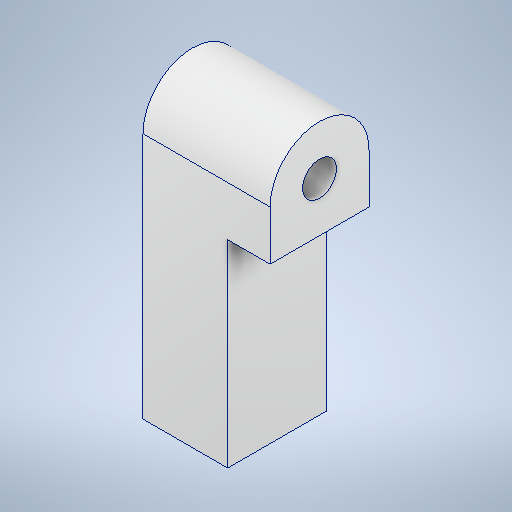
# Autodesk Inventor part: Molde
Saved by Autodesk Inventor 2025.1 (Build 291241000, 241)
## iProperties
Created: 2025-01-29
Part Number: Molde
Material: Aluminum 6061
Document SubType Name: Modeling
Designer: yovan
Mass: 51855.9 g
Surface Area: 6273.43 cm^2
Volume: 19205.9 cm^3
Density: 2.7 g/cm^3
Appearance: Aluminum - Flat
Author: yovan
Autodesk Inventor part; units mm, degrees
ref_plane "YZ Plane" through (0, 0, 0) normal (1, 0, 0) x (0, 1, 0)
ref_plane "XZ Plane" through (0, 0, 0) normal (0, 1, 0) x (-1, 0, 0)
ref_plane "XY Plane" through (0, 0, 0) normal (0, 0, 1) x (1, 0, 0)
sketch "Sketch10" plane through (0, 0, 0) normal (1, 0, 0) x (0, 1, 0)
  line L0 (0, 0) -> (175, 0)
  line L1 (350, -175) -> (350, -175)
  line L2 (175, -350) -> (0, -350)
  line L3 (0, -350) -> (0, 0)
  arc A0 (350, -175) -> (175, 0) centre (175, -175) ccw
  arc A1 (175, -350) -> (350, -175) centre (175, -175) ccw
  point P0 (350, -350)
  point P1 (350, 0)
  dimension "d73" = 350
  dimension "d74" = 350
  dimension "d76" = 175
  constraints: 8 end point, 4 point on circle, 4 point on line, 4 tangent, 2 centre point, 2 parallel, 1 concentric, 1 horizontal, 1 perpendicular
  measures "d73" distance of point (350, -350) L2.end
  measures "d74" distance of point (350, 0) point (350, -350)
  measures "d76" radius of A0
extrude "Extrusion19" add sketch "Sketch10" along normal blind 300
sketch "Sketch11" plane through (300, 0, 0) normal (1, 0, 0) x (0, 0, -1)
  arc A0 (350, 175) -> (0, 175) centre (175, 175) ccw projected
  circle A1 centre (175, 175) radius 60
  point P0 (0, 0)
  dimension "d79" = 120
  constraints: 1 centre point, 1 coincident
  measures "d79" diameter of A1
extrude "Extrusion20" cut sketch "Sketch11" against normal blind 300
sketch "Sketch12" plane through (0, 0, -350) normal (0, -1, 0) x (1, 0, 0)
  line L0 (300, 0) -> (300, 350) projected
  line L1 (0, 350) -> (300, 350)
  line L2 (300, 350) -> (300, 0)
  line L3 (300, 0) -> (0, 0)
  line L4 (0, 0) -> (0, 350)
  constraints: 8 end point, 2 parallel, 1 horizontal, 1 perpendicular
extrude "Extrusion21" add sketch "Sketch12" along normal blind 700
sketch "Sketch13" plane through (300, 0, 0) normal (1, 0, 0) x (0, 0, -1)
  circle A0 centre (175, 175) radius 60 projected
  arc A1 (350, 175) -> (0, 175) centre (175, 175) ccw projected
  arc A2 (350, 175) -> (0, 175) centre (175, 175) ccw
  line L0 (350, 175) -> (350, 0)
  line L1 (350, 0) -> (0, 0)
  line L2 (0, 0) -> (0, 175)
  circle A3 centre (175, 175) radius 60
  constraints: 6 end point, 3 point on circle, 2 centre point, 2 coincident, 1 concentric, 1 parallel
extrude "Extrusion22" add sketch "Sketch13" along normal blind 150
body "Solid3"
